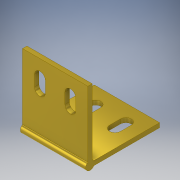
# Autodesk Inventor part: Hinge
Saved by Autodesk Inventor 2018 (Build 220112000, 112)
## iProperties
Created: 2018-02-19
Part Number: Hinge
Material: Generic
Document SubType Name: Modeling
Designer: Melda
Density: 1 g/cm^3
Appearance: Metal 2400F Hot
Author: Melda
Autodesk Inventor part; units mm, degrees
ref_plane "YZ Plane" through (0, 0, 0) normal (1, 0, 0) x (0, 1, 0)
ref_plane "XZ Plane" through (0, 0, 0) normal (0, 1, 0) x (-1, 0, 0)
ref_plane "XY Plane" through (0, 0, 0) normal (0, 0, 1) x (1, 0, 0)
sketch "Sketch1" plane through (0, 0, 0) normal (1, 0, 0) x (0, 1, 0)
  line L0 (1.7321, 1) -> (32, 1)
  line L1 (32, 1) -> (32, -1)
  line L2 (32, -1) -> (1.7321, -1)
  line L3 (1.7321, 1) -> (32, 1)
  line L4 (32, 1) -> (32, -1)
  line L5 (32, -1) -> (1.7321, -1)
  line L6 (1, -1.7273) -> (1, -31.9952)
  line L7 (1, -31.9952) -> (-1, -31.9952)
  line L8 (-1, -31.9952) -> (-1, -1.7273)
  arc A0 (1, -1.7321) -> (1.7321, -1) centre (0, 0) ccw
  arc A1 (1.7321, 1) -> (-1, -1.7321) centre (0, 0) ccw
  dimension "d6" = 2
  dimension "d8" = 30.2679
  dimension "d9" = 30.2679
  dimension "d33" = 2
  constraints: 18 end point, 6 point on circle, 3 parallel, 3 perpendicular, 2 centre point, 2 horizontal, 2 point on line, 1 coincident
  measures "d6" distance of L6.end L7.end
  measures "d8" distance of L1.end L2.end
  measures "d9" distance of L6.start L6.end
  measures "d33" radius of A1
extrude "Extrusion1" add sketch "Sketch1" along normal blind 30
sketch "Sketch2" plane through (0, 1, -1.7321) normal (0, 1, 0) x (1, 0, 0)
  line L0 (8, 22.7632) -> (8, 17.7632) construction
  line L1 (10.5, 22.7632) -> (10.5, 17.7632)
  line L2 (5.5, 17.7632) -> (5.5, 22.7632)
  arc A0 (10.5, 22.7632) -> (5.5, 22.7632) centre (8, 22.7632) ccw
  arc A1 (5.5, 17.7632) -> (10.5, 17.7632) centre (8, 17.7632) ccw
  line L3 (22, 22.7632) -> (22, 17.7632) construction
  line L4 (24.5, 22.7632) -> (24.5, 17.7632)
  line L5 (19.5, 17.7632) -> (19.5, 22.7632)
  arc A2 (24.5, 22.7632) -> (19.5, 22.7632) centre (22, 22.7632) ccw
  arc A3 (19.5, 17.7632) -> (24.5, 17.7632) centre (22, 17.7632) ccw
  line L6 (0, 30.2632) -> (30, 30.2632) projected
  line L7 (30, 30.2632) -> (30, 0) projected
  line L8 (0, 30.2632) -> (0, 0) projected
  point P0 (0, -1.7321)
  point P1 (8, 20.2632)
  point P2 (22, 20.2632)
  dimension "d12" = 5
  dimension "d13" = 10
  dimension "d14" = 5
  dimension "d15" = 10
  dimension "d16" = 10
  dimension "d17" = 10
  dimension "d18" = 8
  dimension "d19" = 8
  constraints: 16 end point, 8 point on circle, 8 tangent, 4 centre point, 2 midpoint, 2 parallel, 2 vertical
  measures "d12" distance between parallel lines of L2 L1
  measures "d14" distance between parallel lines of L5 L4
  measures "d16" distance from line of point (8, 20.263) L6
  measures "d17" distance from line of L6 point (22, 20.263)
  measures "d18" distance from line of L7 point (22, 20.263)
  measures "d19" distance from line of L8 point (8, 20.263)
extrude "Extrusion2" cut sketch "Sketch2" against normal blind 10
sketch "Sketch3" plane through (0, 1.7321, -1) normal (0, 0, -1) x (-1, 0, 0)
  line L0 (-5.5, -0.7321) -> (-10.5, -0.7321) projected
  line L1 (-10.5, -0.7321) -> (-5.5, -0.7321) projected
  line L2 (-19.5, -0.7321) -> (-24.5, -0.7321) projected
  line L3 (-24.5, -0.7321) -> (-19.5, -0.7321) projected
  line L4 (0, -0.7321) -> (-30, -0.7321) projected
  line L5 (0, -0.7321) -> (-30, -0.7321) projected
  line L6 (0, 0) -> (0, 30.2679) projected
  line L7 (0, 30.2679) -> (-30, 30.2679) projected
  line L8 (-30, 0) -> (-30, 30.2679) projected
  line L9 (0, 0) -> (-30, 0) projected
  line L10 (-5.5, -0.7321) -> (-10.5, -0.7321) projected
  line L11 (-10.5, -0.7321) -> (-5.5, -0.7321) projected
  line L12 (-19.5, -0.7321) -> (-24.5, -0.7321) projected
  line L13 (-24.5, -0.7321) -> (-19.5, -0.7321) projected
  line L14 (0, -0.7321) -> (-30, -0.7321) projected
  line L15 (0, -0.7321) -> (-30, -0.7321) projected
  line L16 (-5.5, -0.7321) -> (-10.5, -0.7321) projected
  line L17 (-10.5, -0.7321) -> (-5.5, -0.7321) projected
  line L18 (-19.5, -0.7321) -> (-24.5, -0.7321) projected
  line L19 (-24.5, -0.7321) -> (-19.5, -0.7321) projected
  line L20 (0, -0.7321) -> (-30, -0.7321) projected
  line L21 (0, -0.7321) -> (-30, -0.7321) projected
  line L22 (-5.5, -0.7321) -> (-10.5, -0.7321) projected
  line L23 (-10.5, -0.7321) -> (-5.5, -0.7321) projected
  line L24 (-19.5, -0.7321) -> (-24.5, -0.7321) projected
  line L25 (-24.5, -0.7321) -> (-19.5, -0.7321) projected
  line L26 (0, -0.7321) -> (-30, -0.7321) projected
  line L27 (0, -0.7321) -> (-30, -0.7321) projected
  line L28 (-22, 17.7679) -> (-22, 22.7679) construction
  line L29 (-24.5, 17.7679) -> (-24.5, 22.7679)
  line L30 (-19.5, 22.7679) -> (-19.5, 17.7679)
  arc A0 (-24.5, 17.7679) -> (-19.5, 17.7679) centre (-22, 17.7679) ccw
  arc A1 (-19.5, 22.7679) -> (-24.5, 22.7679) centre (-22, 22.7679) ccw
  line L31 (-8, 17.7679) -> (-8, 22.7679) construction
  line L32 (-10.5, 17.7679) -> (-10.5, 22.7679)
  line L33 (-5.5, 22.7679) -> (-5.5, 17.7679)
  arc A2 (-10.5, 17.7679) -> (-5.5, 17.7679) centre (-8, 17.7679) ccw
  arc A3 (-5.5, 22.7679) -> (-10.5, 22.7679) centre (-8, 22.7679) ccw
  point P0 (0, -1.7321)
  point P1 (-22, 20.2679)
  point P2 (-8, 20.2679)
  dimension "d23" = 10
  dimension "d24" = 5
  dimension "d25" = 10
  dimension "d26" = 8
  dimension "d27" = 10
  dimension "d28" = 5
  dimension "d29" = 8
  dimension "d30" = 10
  constraints: 16 end point, 8 point on circle, 8 tangent, 4 centre point, 2 midpoint, 2 parallel, 2 vertical
  measures "d24" distance between parallel lines of L30 L29
  measures "d25" distance from line of L7 point (-22, 20.268)
  measures "d26" distance from line of L8 point (-22, 20.268)
  measures "d28" distance between parallel lines of L33 L32
  measures "d29" distance from line of L6 point (-8, 20.268)
  measures "d30" distance from line of L7 point (-8, 20.268)
extrude "Extrusion3" cut sketch "Sketch3" against normal blind 10 contours L29 A1 L30 A0 | L32 A3 L33 A2
equation "\"d17\" = d16"
equation "\"d19\" = d18"
equation "\"d29\" = d26"
equation "\"d30\" = d25"
body "Solid1"
